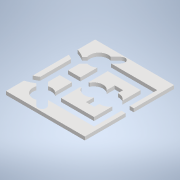
# Autodesk Inventor part: ParteFinalMesaEnsamble
Saved by Autodesk Inventor 2021 (Build 250183000, 183)
## iProperties
Created: 2022-11-05
Part Number: ParteFinalMesaEnsamble
Material: Genérico
Document SubType Name: Modeling
Designer: ivanm
Density: 1 g/cm^3
Appearance: Valor por defecto
Author: ivanm
Autodesk Inventor part; units mm, degrees
ref_plane "YZ Plane" through (0, 0, 0) normal (1, 0, 0) x (0, 1, 0)
ref_plane "XZ Plane" through (0, 0, 0) normal (0, 1, 0) x (-1, 0, 0)
ref_plane "XY Plane" through (0, 0, 0) normal (0, 0, 1) x (1, 0, 0)
sketch "Boceto1" plane through (0, 0, 0) normal (0, 1, 0) x (-1, 0, 0)
  line L0 (-88.8483, 123.588) -> (-88.8483, -136.412)
  line L1 (-88.8483, -136.412) -> (141.1517, -136.412)
  line L2 (141.1517, -136.412) -> (141.1517, 123.588)
  line L3 (141.1517, 123.588) -> (-88.8483, 123.588)
  circle A0 centre (51.468, -121.838) radius 4
  circle A1 centre (51.468, 107.8069) radius 4
  line L4 (66.9242, 84.9845) -> (66.9242, 4.9845)
  line L5 (66.9242, 4.9845) -> (102.9242, 4.9845)
  line L6 (102.9242, 4.9845) -> (102.9242, 54.9845)
  line L7 (126.9242, 54.9845) -> (126.9242, -69.0155)
  line L8 (126.9242, -69.0155) -> (102.9242, -69.0155)
  line L9 (102.9242, -69.0155) -> (102.9242, -19.0155)
  line L10 (102.9242, -19.0155) -> (66.9242, -19.0155)
  line L11 (-77.0758, -99.0155) -> (-77.0758, 84.9845)
  line L12 (-77.0758, 84.9845) -> (66.9242, 84.9845)
  line L13 (-53.0758, -75.0155) -> (42.9242, -75.0155)
  line L14 (42.9242, -75.0155) -> (42.9242, -19.0155)
  line L15 (42.9242, -19.0155) -> (40.111, -19.0155)
  arc A2 (-8.2625, -19.0155) -> (40.111, -19.0155) centre (15.9242, -7.0155) ccw
  line L16 (-8.2625, -19.0155) -> (-53.0758, -19.0155)
  line L17 (-53.0758, -19.0155) -> (-53.0758, -75.0155)
  circle A3 centre (-15.5598, -41.0155) radius 4
  line L18 (42.9242, 60.9845) -> (-53.0758, 60.9845)
  line L19 (-53.0758, 60.9845) -> (-53.0758, 4.9845)
  line L20 (-53.0758, 4.9845) -> (-8.2625, 4.9845)
  arc A4 (40.111, 4.9845) -> (-8.2625, 4.9845) centre (15.9242, -7.0155) ccw
  line L21 (40.111, 4.9845) -> (42.9242, 4.9845)
  line L22 (42.9242, 4.9845) -> (42.9242, 60.9845)
  circle A5 centre (-15.5598, 26.9845) radius 4
  line L23 (-25.5598, -31.5104) -> (-25.5598, -47.0155)
  line L24 (-25.5598, -47.0155) -> (-5.5598, -47.0155)
  line L25 (-5.5598, -47.0155) -> (-5.5598, 32.9845)
  line L26 (-5.5598, 32.9845) -> (-25.5598, 32.9845)
  line L27 (-25.5598, 32.9845) -> (-25.5598, 17.4794)
  arc A6 (-25.5598, 17.4794) -> (-53.4727, 2.9845) centre (-30.5598, -7.0155) ccw
  line L28 (-53.4727, 2.9845) -> (-195.5598, 2.9845)
  line L29 (-195.5598, 2.9845) -> (-195.5598, -17.0155)
  line L30 (-195.5598, -17.0155) -> (-53.4727, -17.0155)
  arc A7 (-53.4727, -17.0155) -> (-25.5598, -31.5104) centre (-30.5598, -7.0155) ccw
  circle A8 centre (-15.5598, 26.9845) radius 4
  circle A9 centre (-15.5598, -41.0155) radius 4
  line L31 (107.8328, -50.9648) -> (92.2599, -66.6277)
  arc A10 (92.2599, -66.6277) -> (59.9496, -99.1245) centre (83.1961, -89.9268) ccw
  line L32 (59.9496, -99.1245) -> (44.3766, -114.7873)
  arc A11 (44.3766, -114.7873) -> (58.5594, -128.8887) centre (51.468, -121.838) ccw
  line L33 (58.5594, -128.8887) -> (74.1323, -113.2259)
  arc A12 (74.1323, -113.2259) -> (106.4427, -80.7291) centre (83.1961, -89.9268) ccw
  line L34 (106.4427, -80.7291) -> (115.9835, -71.1332)
  arc A13 (115.9835, -71.1332) -> (219.4033, -75.1979) centre (171.0539, 12.3369) ccw
  arc A14 (219.4033, -75.1979) -> (209.7334, -57.6909) centre (214.5684, -66.4444) ccw
  arc A15 (121.1609, -50.1986) -> (209.7334, -57.6909) centre (171.0539, 12.3369) ccw
  arc A16 (121.1609, -50.1986) -> (107.8328, -50.9648) centre (114.9242, -58.0155) ccw
  circle A17 centre (51.468, -121.838) radius 4
  circle A18 centre (114.9242, -58.0155) radius 4
  line L35 (107.8328, 36.9338) -> (92.2599, 52.5966)
  arc A19 (107.8328, 36.9338) -> (121.1609, 36.1675) centre (114.9242, 43.9845) ccw
  arc A20 (209.7334, 43.6599) -> (121.1609, 36.1675) centre (171.0539, -26.3679) ccw
  arc A21 (209.7334, 43.6599) -> (219.4033, 61.1668) centre (214.5684, 52.4133) ccw
  arc A22 (219.4033, 61.1668) -> (115.9835, 57.1021) centre (171.0539, -26.3679) ccw
  line L36 (106.4427, 66.698) -> (115.9835, 57.1021)
  arc A23 (106.4427, 66.698) -> (74.1323, 99.1948) centre (83.1961, 75.8957) ccw
  line L37 (58.5594, 114.8576) -> (74.1323, 99.1948)
  arc A24 (58.5594, 114.8576) -> (44.3766, 100.7562) centre (51.468, 107.8069) ccw
  line L38 (59.9496, 85.0934) -> (44.3766, 100.7562)
  arc A25 (59.9496, 85.0934) -> (92.2599, 52.5966) centre (83.1961, 75.8957) ccw
  circle A26 centre (51.468, 107.8069) radius 4
  circle A27 centre (114.9242, 43.9845) radius 4
  line L39 (-27.5598, -33.8483) -> (-27.5598, -49.0155)
  line L40 (-27.5598, -49.0155) -> (-3.5598, -49.0155)
  line L41 (-3.5598, -49.0155) -> (-3.5598, -25.707)
  line L42 (-3.5598, 34.9845) -> (-27.5598, 34.9845)
  line L43 (-27.5598, 34.9845) -> (-27.5598, 19.8173)
  arc A28 (-27.5598, 19.8173) -> (-53.0758, 7.8852) centre (-30.5598, -7.0155) ccw
  arc A29 (74.6524, -115.5394) -> (108.7591, -81.2358) centre (83.1961, -89.9268) ccw
  line L44 (74.6524, -115.5394) -> (59.9777, -130.2988)
  arc A30 (42.9583, -113.3772) -> (59.9777, -130.2988) centre (51.468, -121.838) ccw
  line L45 (42.9583, -113.3772) -> (57.6331, -98.6177)
  arc A31 (91.7398, -64.3142) -> (57.6331, -98.6177) centre (83.1961, -89.9268) ccw
  line L46 (91.7398, -64.3142) -> (106.4146, -49.5547)
  arc A32 (122.4082, -48.6352) -> (106.4146, -49.5547) centre (114.9242, -58.0155) ccw
  arc A33 (122.4082, -48.6352) -> (208.7664, -55.9402) centre (171.0539, 12.3369) ccw
  arc A34 (220.3703, -76.9486) -> (208.7664, -55.9402) centre (214.5684, -66.4444) ccw
  arc A35 (116.2574, -73.6942) -> (220.3703, -76.9486) centre (171.0539, 12.3369) ccw
  line L47 (116.2574, -73.6942) -> (108.7591, -81.2358)
  line L48 (91.7398, 50.2831) -> (106.4146, 35.5236)
  arc A36 (106.4146, 35.5236) -> (122.4082, 34.6041) centre (114.9242, 43.9845) ccw
  line L49 (116.2574, 59.6632) -> (108.7591, 67.2048)
  arc A37 (108.7591, 67.2048) -> (74.6524, 101.5083) centre (83.1961, 75.8957) ccw
  line L50 (74.6524, 101.5083) -> (59.9777, 116.2678)
  arc A38 (59.9777, 116.2678) -> (42.9583, 99.3461) centre (51.468, 107.8069) ccw
  line L51 (42.9583, 99.3461) -> (57.2376, 84.9845)
  line L52 (102.9242, -19.0155) -> (66.9242, -19.0155)
  circle A39 centre (-65.0758, -87.0155) radius 4
  circle A40 centre (-65.0758, 72.9845) radius 4
  line L53 (104.9242, -67.0155) -> (124.9242, -67.0155)
  line L54 (124.9242, -67.0155) -> (124.9242, 52.9845)
  line L55 (124.9242, 52.9845) -> (104.9242, 52.9845)
  line L56 (104.9242, 52.9845) -> (104.9242, 2.9845)
  line L57 (104.9242, 2.9845) -> (64.9242, 2.9845)
  line L58 (64.9242, 2.9845) -> (64.9242, 82.9845)
  line L59 (64.9242, 82.9845) -> (-75.0758, 82.9845)
  line L60 (-75.0758, 82.9845) -> (-75.0758, -97.0155)
  line L61 (-75.0758, -97.0155) -> (64.9242, -97.0155)
  line L62 (64.9242, -97.0155) -> (64.9242, -17.0155)
  line L63 (64.9242, -17.0155) -> (104.9242, -17.0155)
  line L64 (104.9242, -17.0155) -> (104.9242, -67.0155)
  circle A41 centre (114.9242, -58.0155) radius 4
  circle A42 centre (114.9242, 43.9845) radius 4
  line L65 (44.9242, -17.0155) -> (44.9242, -77.0155)
  line L66 (44.9242, -77.0155) -> (-55.0758, -77.0155)
  line L67 (-55.0758, -77.0155) -> (-55.0758, -17.0155)
  line L68 (-55.0758, -17.0155) -> (-6.9887, -17.0155)
  arc A43 (-6.9887, -17.0155) -> (38.8371, -17.0155) centre (15.9242, -7.0155) ccw
  line L69 (38.8371, -17.0155) -> (44.9242, -17.0155)
  line L70 (44.9242, 2.9845) -> (38.8371, 2.9845)
  arc A44 (38.8371, 2.9845) -> (-6.9887, 2.9845) centre (15.9242, -7.0155) ccw
  line L71 (-6.9887, 2.9845) -> (-55.0758, 2.9845)
  line L72 (-55.0758, 2.9845) -> (-55.0758, 62.9845)
  line L73 (-55.0758, 62.9845) -> (44.9242, 62.9845)
  line L74 (44.9242, 62.9845) -> (44.9242, 2.9845)
  line L75 (102.9242, -19.0155) -> (66.9242, -19.0155)
  line L76 (66.9242, -19.0155) -> (66.9242, -68.3809)
  line L77 (-77.0758, -99.0155) -> (-77.0758, 84.9845)
  line L78 (-77.0758, 84.9845) -> (66.9242, 84.9845)
  line L79 (66.9242, 84.9845) -> (66.9242, 4.9845)
  line L80 (66.9242, 4.9845) -> (102.9242, 4.9845)
  line L81 (102.9242, 4.9845) -> (102.9242, 39.0341)
  line L82 (102.9242, -53.0652) -> (102.9242, -19.0155)
  arc A45 (141.1517, 71.1506) -> (116.2574, 59.6632) centre (171.0539, -26.3679) ccw
  arc A46 (141.1517, 45.6727) -> (122.4082, 34.6041) centre (171.0539, -26.3679) ccw
  line L83 (141.1517, 123.588) -> (-88.8483, 123.588)
  line L84 (-88.8483, 123.588) -> (-88.8483, -136.412)
  line L85 (-88.8483, -136.412) -> (141.1517, -136.412)
  line L86 (141.1517, -136.412) -> (141.1517, -85.1816)
  line L87 (126.9242, 37.9483) -> (126.9242, -51.9793)
  arc A47 (66.9242, 54.3498) -> (91.7398, 50.2831) centre (83.1961, 75.8957) ccw
  line L88 (42.9242, 4.9845) -> (40.111, 4.9845)
  arc A48 (40.111, 4.9845) -> (-3.5598, 11.676) centre (15.9242, -7.0155) ccw
  line L89 (-53.0758, 60.9845) -> (42.9242, 60.9845)
  line L90 (42.9242, 60.9845) -> (42.9242, 4.9845)
  line L91 (42.9242, -75.0155) -> (42.9242, -19.0155)
  line L92 (42.9242, -19.0155) -> (40.111, -19.0155)
  line L93 (-53.0758, -75.0155) -> (42.9242, -75.0155)
  line L94 (-3.5598, 11.676) -> (-3.5598, 34.9845)
  line L95 (-53.0758, 7.8852) -> (-53.0758, 60.9845)
  line L96 (-53.0758, -21.9163) -> (-53.0758, -75.0155)
  arc A49 (-3.5598, -25.707) -> (40.111, -19.0155) centre (15.9242, -7.0155) ccw
  arc A50 (-53.0758, -21.9163) -> (-27.5598, -33.8483) centre (-30.5598, -7.0155) ccw
  line L97 (-77.0758, 4.9845) -> (-88.8483, 4.9845)
  line L98 (-88.8483, -19.0155) -> (-77.0758, -19.0155)
  line L99 (57.2376, -99.0155) -> (-77.0758, -99.0155)
  line L100 (57.7718, -99.0155) -> (57.2376, -99.0155)
  line L101 (141.1517, -59.7038) -> (141.1517, 123.588)
  line L102 (141.1517, -85.1816) -> (141.1517, -59.7038)
  point P0 (0, 0)
  point P1 (102.9242, 39.0341)
  point P2 (126.9242, 37.9483)
  point P3 (126.9242, -51.9793)
  point P4 (141.1517, -59.7038)
  point P5 (102.9242, -53.0652)
  point P6 (141.1517, -85.1816)
extrude "Extrusión1" add sketch "Boceto1" along normal blind 10 contours L3 L2 A45 L49 A37 L50 A38 L51 L12 L11 L97 L0 | L98 L11 L99 L45 A30 L44 A29 L47 A35 L2 L1 L0 | L2 A33 L7 A46 | A47 L48 L6 L5 L4 | L76 L10 L9 L46 A31 | L19 L18 L22 L21 A4 L94 L42 L43 A28 | A50 L39 L40 L41 A2 L15 L14 L13 L17
